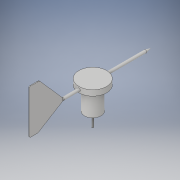
# Autodesk Inventor part: wind_vane
Saved by Autodesk Inventor 2019.4 (Build 234330000, 330)
## iProperties
Created: 2021-02-17
Part Number: wind_vane
Material: Genérico
Document SubType Name: Modeling
Designer: Lattes
Density: 1 g/cm^3
Appearance: Padrão
Author: Lattes
Autodesk Inventor part; units mm, degrees
note: some values were not read from the file. Chosen so that the rebuilt part matches the saved one: edges of "Chanfro1".
ref_plane "YZ Plane" through (0, 0, 0) normal (1, 0, 0) x (0, 1, 0)
ref_plane "XZ Plane" through (0, 0, 0) normal (0, 1, 0) x (-1, 0, 0)
sketch "Esboço1" plane through (0, 0, 0) normal (0, 1, 0) x (-1, 0, 0)
  circle A0 centre (0, 0) radius 15
  dimension "d0" = 30
  constraints: 1 centre point, 1 coincident
  measures "d0" diameter of A0
extrude "Extrusão1" add sketch "Esboço1" along normal blind 30
sketch "Esboço2" plane through (0, 30, 0) normal (0, 1, 0) x (1, 0, 0)
  circle A0 centre (0, 0) radius 2
  dimension "d3" = 4
  constraints: 1 centre point, 1 coincident
  measures "d3" diameter of A0
extrude "Extrusão2" add sketch "Esboço2" along normal blind 1
sketch "Esboço3" plane through (0, 31, 0) normal (0, 1, 0) x (1, 0, 0)
  circle A0 centre (0, 0) radius 25
  dimension "d6" = 50
  constraints: 1 centre point, 1 coincident
  measures "d6" diameter of A0
extrude "Extrusão3" add sketch "Esboço3" along normal blind 10
ref_plane "Plano de trabalho1" through (0, 31, -25) normal (0, 0, 1) x (1, 0, 0)
sketch "Esboço4" plane through (0, 31, -25) normal (0, 0, 1) x (1, 0, 0)
  line L0 (2, 0) -> (-2, 0) projected
  line L1 (0, 0) -> (0, 10)
  line L2 (25, 10) -> (-25, 10) projected
  circle A0 centre (0, 5) radius 2.5
  point P0 (0, -31)
  dimension "d9" = 5
  constraints: 3 midpoint, 2 end point, 1 centre point
  measures "d9" diameter of A0
extrude "Extrusão4" add sketch "Esboço4" along normal blind 80 and the other way blind 70
sketch "Esboço5" plane through (0, 0, 0) normal (1, 0, 0) x (0, 1, 0)
  line L0 (33.5, -95) -> (38.5, -95) projected
  line L1 (36, -95) -> (36, -105)
  line L2 (36, -95) -> (46, -95) construction
  line L3 (36, -105) -> (33.5, -95)
  line L4 (36, -95) -> (33.5, -95)
  point P0 (0, 0)
  dimension "d14" = 10
  dimension "d15" = 90
  constraints: 8 end point, 2 horizontal, 1 midpoint, 1 perpendicular, 1 vertical
  measures "d14" distance of L1.start L1.end
  measures "d15" angle of L1 L2
revolve "Revolução1" add sketch "Esboço5" angle 360 about axis through (0, 36, -95) along (0, 0, -1)
sketch "Esboço6" plane through (0, 0, 0) normal (1, 0, 0) x (0, 1, 0)
  line L0 (38.5, 55) -> (33.5, 55) projected
  line L1 (33.5, 25) -> (33.5, 55) projected
  line L2 (38.5, 25) -> (38.5, 55) projected
  line L3 (33.5, 55) -> (38.5, 55)
  line L4 (6, 113) -> (6, 101.4068)
  line L5 (6.7336, 98.7996) -> (33.5, 55)
  line L6 (8, 115) -> (84, 115)
  line L7 (86, 113) -> (86, 99.2532)
  line L8 (84.312, 95.5075) -> (38.5, 55)
  arc A0 (84.312, 95.5075) -> (86, 99.2532) centre (81, 99.2532) ccw
  arc A1 (6, 101.4068) -> (6.7336, 98.7996) centre (11, 101.4068) ccw
  arc A2 (8, 115) -> (6, 113) centre (8, 113) ccw
  arc A3 (86, 113) -> (84, 115) centre (84, 113) ccw
  point P0 (0, 0)
  point P1 (6, 115)
  point P2 (86, 115)
  point P3 (86, 97)
  dimension "d27" = 80
  dimension "d28" = 18
  dimension "d29" = 5
  dimension "d30" = 2
  constraints: 12 end point, 9 point on line, 8 point on circle, 8 tangent, 4 centre point, 2 equal radius, 2 perpendicular, 1 horizontal
  measures "d27" distance of point (6, 115) point (86, 115)
  measures "d28" distance of point (86, 115) point (86, 97)
  measures "d29" radius of A0
  measures "d30" radius of A2
extrude "Extrusão5" add sketch "Esboço6" along normal mid plane 1.4
chamfer "Chanfro1" distance 1 angle 45 2 edges at (2, 34.5, 55) (-2.5, 36, 55)
sketch "Esboço7" plane through (0, 0, 0) normal (0, -1, 0) x (1, 0, 0)
  circle A0 centre (0, 0) radius 15
  constraints: 1 centre point, 1 coincident
extrude "Extrusão6" add sketch "Esboço7" along normal blind 10
sketch "Esboço8" plane through (0, -10, 0) normal (0, -1, 0) x (1, 0, 0)
  circle A0 centre (0, 0) radius 1.5
  dimension "d39" = 3
  constraints: 1 centre point, 1 coincident
  measures "d39" diameter of A0
extrude "Extrusão7" add sketch "Esboço8" along normal blind 25
thread "Rosca1" size "M3x0.5" class "6g" standard "ANSI Metric M Profile" full length
